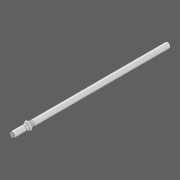
# Autodesk Inventor part: SealantApplicator
Saved by Autodesk Inventor 2020 (Build 240168000, 168)
## iProperties
Created: 2020-01-15
Part Number: SealantApplicator
Material: Generic
Document SubType Name: Modeling
Designer: Isaac Newcomb
Density: 1 g/cm^3
Appearance: Default
Author: Isaac Newcomb
Autodesk Inventor part; units mm, degrees
ref_plane "YZ Plane" through (0, 0, 0) normal (1, 0, 0) x (0, 1, 0)
ref_plane "XZ Plane" through (0, 0, 0) normal (0, 1, 0) x (-1, 0, 0)
ref_plane "XY Plane" through (0, 0, 0) normal (0, 0, 1) x (1, 0, 0)
sketch "Sketch1" plane through (0, 0, 0) normal (0, 1, 0) x (-1, 0, 0)
  line L0 (-3, -22) -> (-3, -180)
  line L1 (-3, -180) -> (0, -180)
  line L2 (0, -180) -> (0, 0)
  line L3 (-5, -18.5) -> (0, -18.5) construction
  line L4 (-5, -18.5) -> (-5, -20.565) construction
  line L5 (-3, -22) -> (-5, -18.5)
  line L6 (-5, -18.5) -> (-3, -15)
  line L7 (-3, -15) -> (-3, 0)
  line L8 (-3, 0) -> (0, 0)
  dimension "d5" = 180
  dimension "d8" = 5
  dimension "d12" = 6
  dimension "d14" = 15
  dimension "d15" = 7
  constraints: 19 end point, 3 perpendicular, 3 vertical, 1 collinear, 1 equal length, 1 horizontal, 1 point on line
  measures "d5" distance of L1.end L2.end
  measures "d8" distance of L3.start L3.end
  measures "d12" diameter of L0 L2
  measures "d14" distance of L6.end L7.end
  measures "d15" distance of L0.start L6.end
revolve "Revolution1" add sketch "Sketch1" angle 360 about axis through (0, 0, -180) along (0, 0, 1)
fillet "Fillet2" radius 5 2 edges at (-3, 0, -22) (-3, 0, -15)
body "Solid1"
